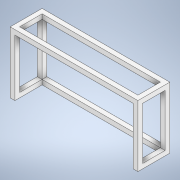
# Autodesk Inventor part: Goal
Saved by Autodesk Inventor 2022 (Build 260153000, 153)
## iProperties
Created: 2022-10-30
Part Number: Goal
Material: 一般
Document SubType Name: Modeling
Designer: Masato Kubotera
Density: 1 g/cm^3
Appearance: 既定
Author: Masato Kubotera
Autodesk Inventor part; units mm, degrees
ref_plane "YZ Plane" through (0, 0, 0) normal (1, 0, 0) x (0, 1, 0)
ref_plane "XZ Plane" through (0, 0, 0) normal (0, 1, 0) x (-1, 0, 0)
ref_plane "XY Plane" through (0, 0, 0) normal (0, 0, 1) x (1, 0, 0)
sketch "スケッチ1" plane through (0, 0, 0) normal (0, 0, 1) x (1, 0, 0)
  line L0 (-300, 1300) -> (300, 1300) construction
  line L1 (300, 1300) -> (300, -1300) construction
  line L2 (300, -1300) -> (-300, -1300) construction
  line L3 (-300, -1300) -> (-300, 1300) construction
  line L4 (-300, 1300) -> (300, -1300) construction
  line L5 (300, 1300) -> (-300, -1300) construction
  line L6 (350, 1350) -> (-325, 1350)
  line L7 (-325, 1350) -> (-325, 1250)
  line L8 (-325, 1250) -> (-225, 1250)
  line L9 (250, 1250) -> (250, -1250)
  line L10 (250, -1250) -> (-225, -1250)
  line L11 (-325, -1250) -> (-325, -1350)
  line L12 (-325, -1350) -> (350, -1350)
  line L13 (350, -1350) -> (350, 1350)
  line L14 (350, 0) -> (-300, 0) construction
  line L15 (-325, 1250) -> (-325, -1250)
  line L16 (-225, -1350) -> (-225, -1250)
  line L17 (250, 1250) -> (250, 1350)
  line L18 (250, -1250) -> (250, -1350)
  line L19 (250, -1250) -> (350, -1250)
  line L20 (250, 1250) -> (350, 1250)
  line L21 (-225, 1250) -> (-225, 1300)
  line L22 (-225, -1250) -> (-225, 1250)
  line L23 (-225, 1300) -> (-225, 1350)
  line L24 (-225, 1250) -> (250, 1250)
  line L25 (-225, -1250) -> (-325, -1250)
  point P0 (0, 0)
  point P1 (0, 0)
  point P2 (0, 0)
  dimension "d0" = 600
  dimension "d1" = 2600
  dimension "d2" = 100
  dimension "d3" = 100
  dimension "d4" = 25
  dimension "d5" = 100
  constraints: 52 end point, 17 perpendicular, 8 point on line, 5 midpoint, 4 parallel, 2 horizontal, 1 coincident, 1 collinear, 5 other
  measures "d0" distance of L0.start L0.end
  measures "d1" distance of L2.end L0.start
  measures "d2" distance between parallel lines of L6 L8
  measures "d3" distance between parallel lines of L13 L9
  measures "d4" distance between parallel lines of L7 L3
  measures "d5" distance between parallel lines of L16 L15
extrude "押し出し1" add sketch "スケッチ1" along normal blind 1300 contours L13 L20 L17 L6 | L17 L24 L21 L23 L6 | L13 L19 L9 L20 | L23 L21 L8 L7 L6 | L13 L12 L18 L19 | L18 L12 L16 L10 | L22 L25 L15 L8 | L16 L12 L11 L25
extrude "押し出し2" cut sketch "スケッチ1" along normal blind 1200 contours L17 L24 L21 L23 L6 | L13 L19 L9 L20 | L9 L10 L22 L24 | L18 L12 L16 L10 | L22 L25 L15 L8
extrude "押し出し3" add sketch "スケッチ1" along normal blind 100 contours L17 L24 L21 L23 L6 | L13 L19 L9 L20 | L18 L12 L16 L10
equation "\"d3\" = d2"
equation "\"d5\" = d2"
